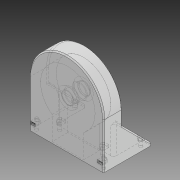
# Autodesk Inventor part: J1_idlebracket
Saved by Autodesk Inventor 2020 (Build 240168000, 168)
## iProperties
Created: 2021-03-20
Part Number: J1_idlebracket
Material: Generic
Document SubType Name: Modeling
Designer: DDeGo
Density: 1 g/cm^3
Appearance: Default
Author: DDeGo
Autodesk Inventor part; units mm, degrees
ref_plane "YZ Plane" through (0, 0, 0) normal (1, 0, 0) x (0, 1, 0)
ref_plane "XZ Plane" through (0, 0, 0) normal (0, 1, 0) x (-1, 0, 0)
ref_plane "XY Plane" through (0, 0, 0) normal (0, 0, 1) x (1, 0, 0)
sketch "Sketch1" plane through (0, 0, 0) normal (0, 0, 1) x (1, 0, 0)
  circle A0 centre (0, 0) radius 47.525
  arc A1 (65, 0) -> (-65, 0) centre (0, 0) ccw
  line L0 (-65, 0) -> (-65, -80)
  line L1 (-65, -80) -> (65, -80)
  line L2 (65, -80) -> (65, 0)
  dimension "d0" = 95.05
  dimension "d2" = 80
  dimension "d43" = 65
  constraints: 6 end point, 2 centre point, 2 coincident, 2 point on circle, 2 tangent, 2 vertical, 1 perpendicular
  measures "d0" diameter of A0
  measures "d2" distance from line of L1 point (0, 0)
  measures "d43" radius of A1
extrude "Extrusion1" add sketch "Sketch1" along normal blind 32.5
sketch "Sketch2" plane through (0, 0, 0) normal (0, 0, -1) x (-1, 0, 0)
  circle A0 centre (0, 0) radius 47.525 projected
  circle A1 centre (0, 0) radius 45.525
  dimension "d5" = 2
  constraints: 1 centre point, 1 coincident
  measures "d5" radial gap between concentric circles of A0 A1
extrude "Extrusion2" add sketch "Sketch2" against normal blind 1
sketch "Sketch3" plane through (0, 0, 32.5) normal (0, 0, 1) x (1, 0, 0)
  arc A0 (65, 0) -> (-65, 0) centre (0, 0) ccw construction
  line L0 (0, 0) -> (0, 55) construction
  circle A1 centre (0, 55) radius 2.6
  circle A2 centre (-52.3081, 16.9959) radius 2.6
  circle A3 centre (-32.3282, -44.4959) radius 2.6
  circle A4 centre (32.3282, -44.4959) radius 2.6
  circle A5 centre (52.3081, 16.9959) radius 2.6
  dimension "d8" = 5.2
  dimension "d9" = 55
  dimension "d12" = 360
  constraints: 5 centre point, 5 coincident, 2 end point, 1 vertical, 16 other
  measures "d8" diameter of A1
  measures "d9" distance of L0.start L0.end
extrude "Extrusion3" cut sketch "Sketch3" against normal through all
sketch "Sketch7" plane through (-65, -80, 0) normal (-1, 0, 0) x (0, 0, 1)
  line L0 (0, 0) -> (32.5, 0) projected
  line L1 (0, 0) -> (-50, 0)
  line L2 (-50, 0) -> (-50, 5)
  line L3 (0, 80) -> (0, 0) projected
  line L4 (-50, 5) -> (0, 55)
  line L5 (0, 0) -> (0, 55)
  dimension "d32" = 50
  dimension "d33" = 5
  dimension "d34" = 135
  constraints: 8 end point, 2 parallel, 1 horizontal, 1 point on line
  measures "d32" distance of L0.start L1.end
  measures "d33" distance of L1.end L2.end
  measures "d34" angle of L2 L4
extrude "Extrusion7" add sketch "Sketch7" against normal blind 15
mirror "Mirror1" about plane through (0, 0, 0) normal (1, 0, 0) of "Extrusion7"
sketch "Sketch5" plane through (-65, -80, 0) normal (0, -1, 0) x (1, 0, 0)
  circle A0 centre (6.5, 26) radius 2.75
  circle A1 centre (123.5, 26) radius 2.75
  circle A2 centre (102.5, 6.5) radius 2.75
  circle A3 centre (27.5, 6.5) radius 2.75
  circle A4 centre (65, 26) radius 2.75
  line L0 (6.5, 26) -> (65, 26) construction
  line L1 (65, 26) -> (123.5, 26) construction
  line L2 (102.5, 6.5) -> (27.5, 6.5) construction
  line L3 (65, 26) -> (65, 6.5) construction
  line L4 (65, 6.5) -> (65, 0) construction
  line L5 (0, 0) -> (130, 0) construction
  line L6 (0, 32.5) -> (130, 32.5) construction
  line L7 (0, 0) -> (0, 32.5) construction
  line L8 (0, -50) -> (15, -50) construction
  line L9 (7.5, -50) -> (7.5, -40) construction
  line L10 (130, -50) -> (115, -50) construction
  line L11 (122.5, -50) -> (122.5, -40) construction
  line L12 (122.5, -40) -> (7.5, -40) construction
  circle A5 centre (7.5, -40) radius 2.75
  circle A6 centre (122.5, -40) radius 2.75
  dimension "d16" = 5.5
  dimension "d17" = 6.5
  dimension "d18" = 6.5
  dimension "d19" = 6.5
  dimension "d37" = 10
  dimension "d59" = 75
  constraints: 16 end point, 7 centre point, 6 equal radius, 4 vertical, 3 horizontal, 3 midpoint, 2 coincident, 1 collinear, 1 perpendicular
  measures "d16" diameter of A0
  measures "d17" distance between parallel lines of L5 L2
  measures "d18" distance between parallel lines of L6 L0
  measures "d19" distance from line of L7 L0.start
  measures "d37" distance of L9.start L9.end
  measures "d59" distance of L2.start L2.end
extrude "Extrusion4" cut sketch "Sketch5" against normal blind 18 contours A0 | A1 | A2 | A3 | A5 | A6
ref_plane "Work Plane1" through (-65, -65, 0) normal (0, -1, 0) x (1, 0, 0)
sketch "Sketch6" plane through (-65, -65, 0) normal (0, -1, 0) x (1, 0, 0)
  circle A0 centre (123.5, 26) radius 2.75 projected
  circle A1 centre (27.5, 6.5) radius 2.75 projected
  line L0 (123.5, 30.7343) -> (127.6, 28.3671) construction
  line L1 (127.6, 28.3671) -> (127.6, 23.6329)
  line L2 (127.6, 23.6329) -> (123.5, 21.2657)
  line L3 (123.5, 21.2657) -> (119.4, 23.6329)
  line L4 (119.4, 23.6329) -> (119.4, 28.3671)
  line L5 (119.4, 28.3671) -> (123.5, 30.7343) construction
  circle A2 centre (27.5, 6.5) radius 2.75 projected
  line L6 (27.5, 1.7657) -> (23.4, 4.1329) construction
  line L7 (23.4, 4.1329) -> (23.4, 8.8671)
  line L8 (23.4, 8.8671) -> (27.5, 11.2343)
  line L9 (27.5, 11.2343) -> (31.6, 8.8671)
  line L10 (31.6, 8.8671) -> (31.6, 4.1329)
  line L11 (31.6, 4.1329) -> (27.5, 1.7657) construction
  circle A3 centre (102.5, 6.5) radius 2.75 projected
  line L12 (102.5, 1.7657) -> (98.4, 4.1329) construction
  line L13 (98.4, 4.1329) -> (98.4, 8.8671)
  line L14 (98.4, 8.8671) -> (102.5, 11.2343)
  line L15 (102.5, 11.2343) -> (106.6, 8.8671)
  line L16 (106.6, 8.8671) -> (106.6, 4.1329)
  line L17 (106.6, 4.1329) -> (102.5, 1.7657) construction
  circle A4 centre (6.5, 26) radius 2.75 projected
  line L18 (6.5, 21.2657) -> (2.4, 23.6329)
  line L19 (2.4, 23.6329) -> (2.4, 28.3671)
  line L20 (2.4, 28.3671) -> (6.5, 30.7343) construction
  line L21 (6.5, 30.7343) -> (10.6, 28.3671) construction
  line L22 (10.6, 28.3671) -> (10.6, 23.6329)
  line L23 (10.6, 23.6329) -> (6.5, 21.2657)
  line L24 (127.6, 28.3671) -> (127.6, 36.5137)
  line L25 (127.6, 36.5137) -> (119.4, 36.5137)
  line L26 (119.4, 36.5137) -> (119.4, 28.3671)
  line L27 (106.6, 4.1329) -> (106.6, -4.3085)
  line L28 (106.6, -4.3085) -> (98.4, -4.3085)
  line L29 (98.4, -4.3085) -> (98.4, 4.1329)
  line L30 (31.6, 4.1329) -> (31.6, -4.965)
  line L31 (31.6, -4.965) -> (23.4, -4.965)
  line L32 (23.4, -4.965) -> (23.4, 4.1329)
  line L33 (17.475, 1) -> (112.525, 1) projected
  line L34 (10.6, 28.3671) -> (10.6, 34.5607)
  line L35 (10.6, 34.5607) -> (2.4, 34.5607)
  line L36 (2.4, 34.5607) -> (2.4, 28.3671)
  circle A5 centre (122.5, -40) radius 2.75 projected
  circle A6 centre (122.5, -40) radius 2.75 projected
  circle A7 centre (7.5, -40) radius 2.75 projected
  line L37 (122.5, -44.7343) -> (118.4, -42.3671)
  line L38 (118.4, -42.3671) -> (118.4, -37.6329)
  line L39 (118.4, -37.6329) -> (122.5, -35.2657)
  line L40 (122.5, -35.2657) -> (126.6, -37.6329)
  line L41 (126.6, -37.6329) -> (126.6, -42.3671)
  line L42 (126.6, -42.3671) -> (122.5, -44.7343)
  line L43 (7.5, -44.7343) -> (3.4, -42.3671)
  line L44 (3.4, -42.3671) -> (3.4, -37.6329)
  line L45 (3.4, -37.6329) -> (7.5, -35.2657)
  line L46 (7.5, -35.2657) -> (11.6, -37.6329)
  line L47 (11.6, -37.6329) -> (11.6, -42.3671)
  line L48 (11.6, -42.3671) -> (7.5, -44.7343)
  point P0 (65, 0)
  point P1 (65, 26)
  point P2 (31.6, 1)
  point P3 (23.4, 1)
  point P4 (106.6, 1)
  point P5 (98.4, 1)
  dimension "d23" = 8.2
  constraints: 96 end point, 10 vertical, 6 coincident, 5 perpendicular, 3 collinear, 2 equal length, 78 other
  measures "d23" distance between parallel lines of L4 L1
extrude "Extrusion5" cut sketch "Sketch6" along normal blind 4.5
extrude "Extrusion6" cut sketch "Sketch6" against normal blind 20.75 contours L37 L38 L39 L40 L41 L42 | L43 L44 L45 L46 L47 L48
chamfer "Chamfer1" distance 2 angle 45 10 edges at (0, 65, 32.5) (-65, -40, 32.5) (65, -40, 32.5) (0, 65, 0) (-65, -12.5, 0) (65, -12.5, 0) (-65, -50, -25) (-50, -50, -25) (50, -50, -25) (65, -50, -25)
fillet "Fillet2" radius 5 4 edges at (-50, -53.9142, 0) (50, -53.9142, 0) (57.5, -25, 0) (-57.5, -25, 0)
sketch "Sketch10" plane through (0, 0, 0) normal (1, 0, 0) x (0, 1, 0)
  line L0 (-47.525, 1) -> (47.525, 1) construction
  line L1 (-47.525, 32.5) -> (47.525, 32.5) construction
  line L2 (-47.525, 32.5) -> (-47.525, 1) construction
  line L3 (45.525, 0) -> (-45.525, 0) construction
  line L4 (-47.525, 1) -> (47.525, 1) construction
  line L5 (-47.525, 1) -> (-47.525, 0)
  line L6 (-47.525, 0) -> (-45.525, 0)
  line L7 (0, 32.5) -> (0, 0) construction
  line L8 (-10.1, 0) -> (-10.1, 2)
  line L9 (-10.1, 2) -> (-11.1, 2)
  line L10 (-11.1, 2) -> (-11.1, 9)
  line L11 (0, 30.5) -> (0, 32.5)
  line L12 (0, 30.5) -> (-10.1, 30.5)
  line L13 (-11.1, 23) -> (-13.1, 23)
  line L14 (-13.1, 23) -> (-17.1415, 30)
  line L15 (-17.1415, 30) -> (-47.525, 30)
  line L16 (-47.525, 32.5) -> (47.525, 32.5) construction
  line L17 (-47.525, 30) -> (-47.525, 32.5)
  line L18 (-10.1, 30.5) -> (-10.1, 30)
  line L19 (-10.1, 30) -> (-11.1, 30)
  line L20 (-11.1, 30) -> (-11.1, 23)
  line L21 (-11.1, 9) -> (-13.1, 9)
  line L22 (-13.1, 9) -> (-16.8528, 2.5)
  line L23 (-16.8528, 2.5) -> (-47.525, 2.5)
  line L24 (-47.525, 2.5) -> (-47.525, 1)
  line L25 (-45.525, 0) -> (-10.1, 0)
  line L26 (-47.525, 32.5) -> (0, 32.5)
  dimension "d44" = 11.1
  dimension "d45" = 1
  dimension "d46" = 0.5
  dimension "d47" = 2
  dimension "d48" = 2.5
  dimension "d49" = 7
  dimension "d51" = 2
  dimension "d52" = 120
  dimension "d53" = 2
  dimension "d54" = 11.1
  dimension "d55" = 2.5
  dimension "d56" = 120
  constraints: 42 end point, 8 perpendicular, 5 vertical, 4 point on line, 3 collinear, 3 equal length, 2 horizontal, 1 midpoint, 1 parallel
  measures "d44" distance between parallel lines of L20 L7
  measures "d45" distance of L18.end L19.end
  measures "d46" distance of L12.end L18.end
  measures "d47" distance between parallel lines of L1 L12
  measures "d48" distance between parallel lines of L1 L15
  measures "d49" distance of L19.end L13.start
  measures "d51" distance of L13.start L13.end
  measures "d52" angle of L13 L14
  measures "d53" distance of L8.start L8.end
  measures "d54" distance between parallel lines of L7 L10
  measures "d55" distance between parallel lines of L25 L23
  measures "d56" angle of L21 L22
revolve "Revolution1" add sketch "Sketch10" angle 360 about axis through (0, 0, 32.5) along (0, 0, -1)
sketch "Sketch12" plane through (0, 0, 32.5) normal (0, 0, 1) x (1, 0, 0)
  circle A0 centre (-52.3081, 16.9959) radius 2.6 projected
  circle A1 centre (0, 55) radius 2.6 projected
  circle A2 centre (52.3081, 16.9959) radius 2.6 projected
  circle A3 centre (32.3282, -44.4959) radius 2.6 projected
  circle A4 centre (-32.3282, -44.4959) radius 2.6 projected
  point P0 (0, 0)
extrude "Extrusion8" add sketch "Sketch12" against normal up to surface (32.5 mm away)
sketch "Sketch11" plane through (0, 0, 30) normal (0, 0, -1) x (-1, 0, 0)
  circle A0 centre (0, 0) radius 47.525 construction
  line L0 (63, -80) -> (-63, -80) projected
  line L1 (-27.5, -38.7605) -> (27.5, -38.7605)
  line L2 (27.5, -38.7605) -> (27.5, -80)
  line L3 (27.5, -80) -> (-27.5, -80)
  line L4 (-27.5, -80) -> (-27.5, -38.7605)
  circle A1 centre (0, 0) radius 47.525 construction
  dimension "d58" = 55
  constraints: 8 end point, 2 parallel, 1 horizontal, 1 perpendicular, 1 point on circle, 1 point on line, 2 other
  measures "d58" distance of L1.start L1.end
extrude "Extrusion9" cut sketch "Sketch11" along normal up to surface (27.5 mm away)
equation "\"d18\" = d17"
equation "\"d19\" = d17"
equation "\"d54\" = d44"
equation "\"d56\" = d52"
body "Solid1"
